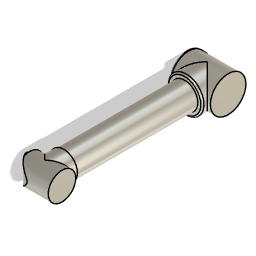
Link4 v19 (Autodesk Fusion 360 design; units mm, degrees)
Autodesk Fusion 360 part; units mm, degrees
sketch "Boceto1" plane through (0, 0, 0) normal (0, 0, 1) x (1, 0, 0)
  circle A0 centre (0, 0) radius 58
  dimension "d1" = 116
  constraint coincident A0.centre origin
  measures "d1" diameter of A0
extrude "Extruir1" add sketch "Boceto1" along normal blind 136
sketch "Boceto2" plane through (0, 0, 0) normal (1, 0, 0) x (0, 0, -1)
  circle A0 centre (-68, 0) radius 58
  line L0 (0, 58) -> (0, -58)
  dimension "d4" = 116
  dimension "d5" = 68
  measures "d4" diameter of A0
  measures "d5" distance of A0.centre L0
extrude "Extruir2" add sketch "Boceto2" along normal blind 74
sketch "Boceto3" plane through (74, 0, 0) normal (1, 0, 0) x (0, 0, -1)
  circle A0 centre (-68, 0) radius 58
  circle A1 centre (-68, 0) radius 43
  circle A2 centre (-68, 0) radius 30
  dimension "d8" = 86
  dimension "d26" = 60
  constraint concentric A0 A1
  constraint concentric A1 A2
  measures "d8" diameter of A1
  measures "d26" diameter of A2
extrude "Extruir3" add sketch "Boceto3" along normal blind 395 contours A1 | A2
sketch "Boceto4" plane through (469, 0, 0) normal (1, 0, 0) x (0, 0, -1)
  circle A0 centre (-68, 0) radius 43
  circle A1 centre (-68, 0) radius 45
  dimension "d11" = 90
  constraint concentric A0 A1
  measures "d11" diameter of A1
extrude "Extruir4" add sketch "Boceto4" along normal blind 62 contours A0 | A1
ref_plane "PlanoDeObra1" through (0, 0, 68) normal (0, 0, 1) x (1, 0, 0)
sketch "Boceto5" plane through (0, 0, 68) normal (0, 0, 1) x (1, 0, 0)
  circle A0 centre (531, 0) radius 45
  point P0 (469, 0)
  dimension "d14" = 90
  dimension "d15" = 62
  measures "d14" diameter of A0
  measures "d15" distance of A0.centre P0
extrude "Extruir5" add sketch "Boceto5" along normal mid plane 113
fillet "Empalme1" radius 7 1 edges at (-54.075, -20.9737, 0)
fillet "Empalme2" radius 5 1 edges at (74, -20.9737, 122.075)
fillet "Empalme3" radius 7 1 edges at (489.0453, 16.2727, 11.5)
sketch "Sketch6" plane through (0, 0, 0) normal (0, 1, 0) x (1, 0, 0)
  spline S0 degree 5 poles (20, 0) (10.8406, 0) (-5.724, -0.5954) (-25.3136, -3.2735) (-42.3808, -10.2968) (-53.7584, -25.5601) (-58.1008, -44.8558) (-59.6546, -64.9283) (-60, -81.1663) (-60, -90) knots 0 0 0 0 0 0 0.2 0.4 0.6 0.8 1 1 1 1 1 1
  line L0 (-60, -70) -> (-60, -110)
  line L1 (40, 0) -> (0, 0)
  line L2 (-60, -90) -> (-60, 0)
  line L3 (-60, 0) -> (20, 0)
  constraint midpoint S0.end L0
  constraint midpoint S0.start L1
  constraint perpendicular L0 L3
extrude "Extrude6" cut sketch "Sketch6" along normal through all and the other way through all
sketch "Sketch7" plane through (0, 0, 0) normal (0, 1, 0) x (1, 0, 0)
  spline S0 degree 5 poles (510, -10) (516.0702, -9.9405) (527.3406, -10.5077) (541.6385, -13.4153) (556.1114, -20.8563) (568.436, -34.2402) (574.4757, -47.1394) (576.8208, -57.7833) (577.3422, -65.3075) (577.3422, -69.1768) knots 0 0 0 0 0 0 0.2 0.4 0.6 0.8 1 1 1 1 1 1
  line L0 (577.3422, -59.1768) -> (577.3422, -79.1768)
  line L1 (493.7236, -10.1596) -> (526.2764, -9.8404)
  line L2 (577.3422, -69.1768) -> (577.3422, -10)
  line L3 (577.3422, -10) -> (510, -10)
  constraint midpoint S0.end L0
  constraint midpoint S0.start L1
  constraint perpendicular L0 L3
extrude "Extrude7" cut sketch "Sketch7" along normal through all and the other way through all contours S0 L0 L2 L3
extrude "Extrude8" cut sketch "Boceto3" along normal blind 395 contours A2
move_body "Desplazar1" bodies 1 to x (0.017452, 0.999848, 0) y (0, 0, 1) z (0.999848, -0.017452, 0) at (-56.9913, -0.0006, 57.9953)
move_body "Desplazar2" bodies 1 to x (1, 0, 0) y (0, 1, 0) z (0, 0, 1) at (0, 50, -50)
move_body "Desplazar3" bodies 1 to x (0.034899, 0.999391, 0) y (0.999391, -0.034899, 0) z (0, 0, -1) at (-110.8657, 114.8048, 15.9907)
move_body "Desplazar4" bodies 1 to x (0.999848, 0.017452, 0) y (-0.017452, 0.999848, 0) z (0, 0, 1) at (63.8552, -190.9719, -8)
sketch "Sketch8" plane through (0, 0, 0) normal (0, 0, 1) x (1, 0, 0)
  line L0 (0, 0) -> (-59.45, 0)
  point P0 (56.55, 0)
  dimension "d32" = 59.45
  dimension "d33" = 116
  constraint coincident L0.start origin
  constraint horizontal L0
  measures "d32" distance of L0.start L0.end
  measures "d33" distance of L0.end P0
sketch "Sketch9" plane through (0, 0.0253, 0) normal (0, 1, 0) x (-1, 0, 0)
  circle A0 centre (0, -0.0047) radius 58
sketch "Sketch10" plane through (0, 0, 0) normal (0, 0, 1) x (1, 0, 0)
  point P0 (486, -11.4747)
  dimension "d34" = 11.4747
  measures "d34" vertical distance of P0 origin
sketch "Sketch11" plane through (0, 0.0253, 0) normal (0, 1, 0) x (-1, 0, 0)
  circle A0 centre (0, -0.0047) radius 58
sketch "Sketch12" plane through (0, -11.4747, 0) normal (0, 1, 0) x (-1, 0, 0)
  circle A0 centre (-531, -0.0047) radius 45
  line L0 (-531, -0.0047) -> (0, 0)
  dimension "d35" = 531
  constraint coincident A0.centre L0.start
  constraint coincident L0.end origin
  measures "d35" horizontal distance of A0.centre L0.end
